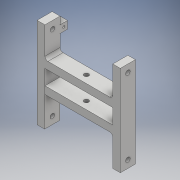
# Autodesk Inventor part: SoporteOjos
Saved by Autodesk Inventor 2017 SP1 (Build 210196100, 196)
## iProperties
Part Number: SoporteOjos
Material: Genérico
Document SubType Name: Modeling
Designer: Juan
Density: 1 g/cm^3
Appearance: Valor por defecto
Author: Juan
Autodesk Inventor part; units mm, degrees
sketch "Boceto1" plane through (0, 0, 0) normal (0, 1, 0) x (-1, 0, 0)
  line L0 (0, 60) -> (0, 0)
  line L1 (0, 0) -> (-5, 0)
  line L2 (-5, 0) -> (-5.2064, 24.9991)
  line L3 (-5.2064, 24.9991) -> (-50.2064, 24.9991)
  line L4 (-5.2064, 24.9991) -> (39.7936, 24.9991) construction
  line L5 (-50.2064, 24.9991) -> (-50.2064, -0.0009)
  line L6 (-50.2064, -0.0009) -> (-55.2064, -0.0009)
  line L7 (-55.2064, -0.0009) -> (-55.2064, 59.9991)
  line L8 (-55.2064, 59.9991) -> (-50.2064, 59.9991)
  line L9 (-50.2064, 59.9991) -> (-50.2064, 34.9991)
  line L10 (-50.2064, 34.9991) -> (-5.2064, 34.9991)
  line L11 (-5.2064, 34.9991) -> (-5.2064, 59.9991)
  line L12 (-5.2064, 59.9991) -> (0, 60)
  line L13 (-5.2064, 34.9991) -> (-5.2064, 39.9991)
  line L14 (-5.2064, 34.9991) -> (-5.2064, 39.9991)
  line L15 (-5.2064, 39.9991) -> (-50.2064, 39.9991)
  line L16 (-5.2064, 39.9991) -> (39.7936, 39.9991) construction
  line L17 (-50.2064, 39.9991) -> (-50.2064, 34.9991)
  line L18 (-5.2064, 24.9991) -> (-0.2064, 24.9991) construction
  line L19 (-5.2064, 19.9991) -> (-50.2064, 19.9991)
  line L20 (-50.2064, 19.9991) -> (-50.2064, 24.9991)
  line L21 (-5.2064, 24.9991) -> (-5.2064, 19.9991)
  line L22 (-5.2064, 24.9991) -> (-0.2064, 24.9991) construction
  dimension "d0" = 60
  dimension "d1" = 5
  dimension "d2" = 25
  dimension "d3" = 45
  dimension "d4" = 180
  dimension "d5" = 25
  dimension "d6" = 5
  dimension "d7" = 90
  dimension "d8" = 60
  dimension "d9" = 5
  dimension "d10" = 90
  dimension "d11" = 25
  dimension "d12" = 25
  dimension "d13" = 5
  dimension "d14" = 45
  dimension "d15" = 180
  dimension "d16" = 5
  dimension "d18" = 45
  dimension "d30" = 90
  constraints: 46 end point, 8 perpendicular, 5 horizontal, 4 point on line, 3 equal length, 2 collinear, 2 vertical, 1 coincident
  measures "d0" distance of L0.start L0.end
  measures "d1" distance of L0.end L1.end
  measures "d2" distance of L1.end L2.end
  measures "d3" distance of L2.end L3.end
  measures "d4" angle of L3 L4
  measures "d5" distance of L3.end L5.end
  measures "d6" distance of L5.end L6.end
  measures "d7" angle of L5 L6
  measures "d8" distance of L6.end L7.end
  measures "d9" distance of L7.end L8.end
  measures "d10" angle of L7 L8
  measures "d11" distance of L8.end L9.end
  measures "d12" distance of L10.end L11.end
  measures "d13" distance of L10.end L13.end
  measures "d14" distance of L13.end L15.end
  measures "d15" angle of L15 L16
  measures "d16" distance of L2.end L19.start
  measures "d18" distance of L19.start L19.end
  measures "d30" angle of L21 L22
extrude "Extrusión1" add sketch "Boceto1" along normal blind 10
ref_plane "Plano de trabajo1" through (0, 10, 0) normal (0, 1, 0) x (1, 0, 0)
sketch "Boceto2" plane through (0, 10, 0) normal (0, 1, 0) x (1, 0, 0)
  line L0 (5.2064, -59.9991) -> (5.2064, -39.9991) construction
  line L1 (5.2064, -39.9991) -> (5.2064, -34.9991) construction
  line L2 (5.2064, -34.9991) -> (50.2064, -34.9991)
  line L3 (50.2064, -34.9991) -> (50.2064, -24.9991)
  line L4 (50.2064, -24.9991) -> (5.2064, -24.9991)
  line L5 (5.2064, -24.9991) -> (5.2064, -34.9991)
  point P0 (0, 0)
  dimension "d22" = 5
  dimension "d23" = 45
  dimension "d24" = 10
  constraints: 10 end point, 2 parallel, 1 horizontal, 1 perpendicular, 1 vertical
  measures "d22" distance of L0.end L1.end
  measures "d23" distance of L4.end L3.end
  measures "d24" distance of L3.end L2.end
extrude "Extrusión2" cut sketch "Boceto2" against normal blind 10
fillet "Empalme1" radius 2 1 edges at (5.2064, 5, 39.9991)
fillet "Empalme2" radius 2 1 edges at (50.2064, 5, 39.9991)
fillet "Empalme3" radius 2 1 edges at (50.2064, 5, 19.9991)
ref_plane "Plano de trabajo2" through (50.2064, 10, 34.9991) normal (0, 0, -1) x (-1, 0, 0)
sketch "Boceto3" plane through (50.2064, 10, 34.9991) normal (0, 0, -1) x (-1, 0, 0)
  line L0 (0, 0) -> (45, 0) construction
  line L1 (45, 0) -> (0, -10) construction
  line L2 (45, -10) -> (0, 0) construction
  line L3 (22.5, -5) -> (22.5, 0) construction
  point P0 (50.2064, -10)
  constraints: 6 end point, 2 midpoint
hole "Agujero1" at (27.7064, 5, 34.9991) direction (0, 0, 1) diameter 3 end through all
ref_plane "Plano de trabajo3" through (5.2064, 10, 24.9991) normal (0, 0, 1) x (1, 0, 0)
sketch "Boceto4" plane through (5.2064, 10, 24.9991) normal (0, 0, 1) x (1, 0, 0)
  line L0 (45, 0) -> (45, -10) construction
  line L1 (0, -10) -> (45, 0) construction
  line L2 (45, -10) -> (0, -10) construction
  line L3 (0, 0) -> (45, -10) construction
  line L4 (22.5, -5) -> (23.0086, 0) construction
  line L5 (0, 0) -> (45, 0) construction
  point P0 (-5.2064, -10)
  constraints: 6 end point, 1 midpoint, 1 point on line
hole "Agujero2" at (27.7064, 5, 24.9991) direction (0, 0, -1) diameter 3 end through all
ref_plane "Plano de trabajo4" through (0, 10, 0) normal (0, 1, 0) x (1, 0, 0)
sketch "Boceto5" plane through (0, 10, 0) normal (0, 1, 0) x (1, 0, 0)
  line L0 (0, 0) -> (0, -60) construction
  line L1 (0, -60) -> (0, -55) construction
  line L2 (5.2064, -59.9991) -> (5.2064, -41.9991) projected
  line L3 (0, -55) -> (5.2064, -55)
  line L4 (5.2064, -55) -> (5.2064, -50)
  line L5 (5.2064, -50) -> (0, -50)
  line L6 (0, -50) -> (0, -55)
  line L7 (0, -50) -> (0, -19) construction
  line L8 (0, -19) -> (5.2064, -19)
  line L9 (5.2064, -19) -> (5.2064, -14)
  line L10 (5.2064, -14) -> (0, -14)
  line L11 (0, -14) -> (0, -19)
  dimension "d48" = 5
  dimension "d49" = 5
  dimension "d50" = 31
  dimension "d51" = 5
  constraints: 20 end point, 4 parallel, 3 point on line, 2 horizontal, 2 perpendicular
  measures "d48" distance of L0.end L1.end
  measures "d49" distance of L4.end L3.end
  measures "d50" distance of L5.end L7.end
  measures "d51" distance of L9.end L8.end
extrude "Extrusión3" add sketch "Boceto5" along normal blind 5
sketch "Boceto6" plane through (0, 0, 0) normal (-1, 0, 0) x (0, 0, 1)
  line L0 (59.9991, 10) -> (55, 10) construction
  line L1 (50, 10) -> (50, 15) construction
  line L2 (55, 10) -> (50, 15) construction
  line L3 (50, 10) -> (52.5, 12.5) construction
  line L4 (19, 10) -> (14, 10) construction
  line L5 (14, 15) -> (19, 15) construction
  line L6 (14, 10) -> (19, 15) construction
  line L7 (14, 15) -> (16.5, 12.5) construction
  point P0 (0, 0)
  constraints: 8 end point, 2 midpoint
hole "Agujero3" at (0, 12.5, 16.5) at (0, 12.5, 52.5) direction (1, 0, 0) diameter 1.5 end through all
sketch "Boceto7" plane through (0, 0, 0) normal (-1, 0, 0) x (0, 0, 1)
  line L0 (-0.0009, 0) -> (-0.0009, 10) construction
  line L1 (-0.0009, 10) -> (-0.0009, 5) construction
  line L2 (-0.0009, 5) -> (4.9991, 5) construction
  line L3 (41.9991, 10) -> (59.9991, 10) construction
  line L4 (59.9991, 10) -> (59.9991, 5) construction
  line L5 (59.9991, 0) -> (59.9991, 10) construction
  line L6 (59.9991, 5) -> (54.9991, 5) construction
  point P0 (0, 0)
  dimension "d63" = 5
  dimension "d64" = 5
  constraints: 8 end point, 2 midpoint, 2 perpendicular
  measures "d63" distance of L1.end L2.end
  measures "d64" distance of L4.end L6.end
hole "Agujero4" at (0, 5, 4.9991) at (0, 5, 54.9991) direction (1, 0, 0) diameter 3 end through all
